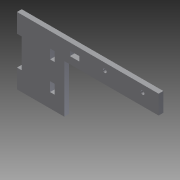
# Autodesk Inventor part: side 1
Saved by Autodesk Inventor 2011 (Build 150239000, 239)
## iProperties
Created: 2011-02-20
Part Number: side 1
Document SubType Name: Modeling
Designer: adowning
Density: 1 g/cm^3
Author: adowning
Autodesk Inventor part; units mm, degrees
ref_plane "YZ Plane" through (0, 0, 0) normal (1, 0, 0) x (0, 1, 0)
ref_plane "XZ Plane" through (0, 0, 0) normal (0, 1, 0) x (-1, 0, 0)
ref_plane "XY Plane" through (0, 0, 0) normal (0, 0, 1) x (1, 0, 0)
sketch "Sketch2" plane through (0, 0, 0) normal (0, 0, 1) x (1, 0, 0)
  line L0 (-75.3899, 25.3495) -> (108.7601, 25.3495)
  line L1 (108.7601, 25.3495) -> (108.7601, -0.0505)
  line L2 (108.7601, -0.0505) -> (-18.2399, -0.0505)
  line L3 (-75.3899, 25.3495) -> (-75.3899, -64.8205)
  line L4 (-75.3899, -64.8205) -> (-18.2399, -64.8205)
  line L5 (-18.2399, -64.8205) -> (-18.2399, -0.0505)
  line L6 (-75.3899, 25.3495) -> (-81.7399, 25.3495)
  line L7 (-81.7399, 25.3495) -> (-81.7399, -0.0505)
  line L8 (-81.7399, -0.0505) -> (-75.3899, -0.0505)
  line L9 (-75.3899, -64.8205) -> (-81.7399, -64.8205)
  line L10 (-81.7399, -64.8205) -> (-81.7399, -39.4205)
  line L11 (-81.7399, -39.4205) -> (-75.3899, -39.4205)
  line L12 (108.7601, 25.3495) -> (87.1701, 25.3495)
  line L13 (87.1701, 25.3495) -> (87.1701, 15.8245)
  line L14 (87.1701, 15.8245) -> (36.3701, 15.8245)
  circle A0 centre (36.3701, 15.8245) radius 2.4892
  circle A1 centre (87.1701, 15.8245) radius 2.4892
  line L15 (-18.2399, -64.8205) -> (-18.2399, -45.7705)
  line L16 (-18.2399, -45.7705) -> (-37.2899, -45.7705)
  line L17 (-37.2899, -45.7705) -> (-37.2899, -33.0705)
  line L18 (-37.2899, -33.0705) -> (-30.9399, -33.0705)
  line L19 (-30.9399, -33.0705) -> (-30.9399, -7.6705)
  line L20 (-30.9399, -7.6705) -> (-37.2899, -7.6705)
  line L21 (-37.2899, -7.6705) -> (-37.2899, 5.0295)
  line L22 (-37.2899, 5.0295) -> (-30.9399, 5.0295)
  line L23 (-30.9399, 5.0295) -> (-30.9399, -7.6705)
  line L24 (-30.9399, -33.0705) -> (-30.9399, -45.7705)
  point P0 (0, 0)
  dimension "d5" = 184.15
  dimension "d6" = 25.4
  dimension "d7" = 127
  dimension "d8" = 90.17
  dimension "d9" = 6.35
  dimension "d10" = 25.4
  dimension "d11" = 25.4
  dimension "d12" = 21.59
  dimension "d13" = 9.525
  dimension "d14" = 50.8
  dimension "d15" = 4.9784
  dimension "d16" = 4.9784
  dimension "d17" = 19.05
  dimension "d18" = 19.05
  dimension "d19" = 12.7
  dimension "d20" = 6.35
  dimension "d21" = 25.4
  dimension "d22" = 6.35
  dimension "d23" = 12.7
  constraints: 50 end point, 13 perpendicular, 8 parallel, 5 point on line, 2 centre point, 2 coincident, 1 collinear, 1 horizontal
  measures "d5" distance of L0.start L0.end
  measures "d6" distance of L0.end L1.end
  measures "d7" distance of L1.end L2.end
  measures "d8" distance of L0.start L3.end
  measures "d9" distance of L0.start L6.end
  measures "d10" distance of L6.end L7.end
  measures "d11" distance of L9.end L10.end
  measures "d12" distance of L0.end L12.end
  measures "d13" distance of L12.end L13.end
  measures "d14" distance of L13.end L14.end
  measures "d15" diameter of A0
  measures "d16" diameter of A1
  measures "d17" distance of L4.end L15.end
  measures "d18" distance of L15.end L16.end
  measures "d19" distance of L16.end L17.end
  measures "d20" distance of L17.end L18.end
  measures "d21" distance of L18.end L19.end
  measures "d22" distance of L19.end L20.end
  measures "d23" distance of L20.end L21.end
extrude "Extrusion1" add sketch "Sketch2" along normal blind 6.35
sketch "Sketch3" plane through (0, 0, 6.35) normal (0, 0, 1) x (1, 0, 0)
  line L0 (-81.7399, 25.3495) -> (108.7601, 25.3495) projected
  line L1 (108.7601, 25.3495) -> (2.0801, 25.3495)
  line L2 (2.0801, 25.3495) -> (2.0801, 15.8245)
  line L3 (2.0801, 15.8245) -> (-10.6199, 15.8245)
  line L4 (-10.6199, 15.8245) -> (-10.6199, 9.4745)
  line L5 (-10.6199, 9.4745) -> (2.0801, 9.4745)
  line L6 (2.0801, 9.4745) -> (2.0801, 15.8245)
  point P0 (0, 0)
  dimension "d26" = 106.68
  dimension "d27" = 9.525
  dimension "d28" = 12.7
  dimension "d29" = 6.35
  constraints: 12 end point, 2 parallel, 2 perpendicular, 1 collinear, 1 point on line
  measures "d26" distance of L0.end L1.end
  measures "d27" distance of L1.end L2.end
  measures "d28" distance of L2.end L3.end
  measures "d29" distance of L3.end L4.end
extrude "Extrusion2" cut sketch "Sketch3" against normal blind 25.4
body "Solid1"
